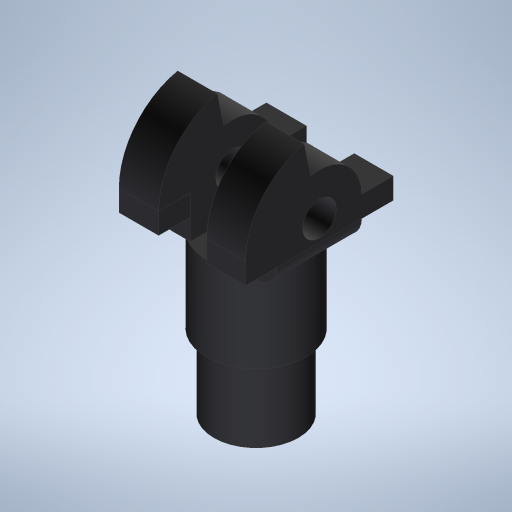
# Autodesk Inventor part: hingejoint2
Saved by Autodesk Inventor 2024 (Build 280153000, 153)
## iProperties
Created: 2024-05-16
Part Number: hingejoint2
Material: Generic
Document SubType Name: Modeling
Designer: maja6
Density: 1 g/cm^3
Appearance: Default
Author: maja6
Autodesk Inventor part; units mm, degrees
ref_plane "YZ Plane" through (0, 0, 0) normal (1, 0, 0) x (0, 1, 0)
ref_plane "XZ Plane" through (0, 0, 0) normal (0, 1, 0) x (-1, 0, 0)
ref_plane "XY Plane" through (0, 0, 0) normal (0, 0, 1) x (1, 0, 0)
sketch "Sketch1" plane through (0, 0, 0) normal (0, 0, 1) x (1, 0, 0)
  circle A0 centre (0, 0) radius 2
  circle A1 centre (0, 0) radius 4
  dimension "d0" = 4
  dimension "d1" = 8
  constraints: 2 centre point, 2 coincident
  measures "d0" diameter of A0
  measures "d1" diameter of A1
extrude "Extrusion1" add sketch "Sketch1" along normal blind 15
sketch "Sketch2" plane through (0, 0, 15) normal (0, 0, 1) x (1, 0, 0)
  circle A0 centre (0, 0) radius 4 projected
  line L0 (0, 4) -> (6, 4)
  line L1 (6, 4) -> (6, -4)
  line L2 (6, -4) -> (0, -4)
  line L3 (0, -4) -> (0, 4)
  line L4 (0, 4) -> (-6, 4)
  line L5 (-6, 4) -> (-6, -4)
  line L6 (-6, -4) -> (0, -4)
  line L7 (0, -4) -> (0, 4)
  dimension "d4" = 6
  dimension "d5" = 6
  constraints: 16 end point, 4 parallel, 2 horizontal, 2 perpendicular, 1 point on line, 1 vertical alignment, 1 other
  measures "d4" distance of L1.end L2.end
  measures "d5" distance of L6.end L5.end
extrude "Extrusion2" add sketch "Sketch2" along normal blind 8
sketch "Sketch3" plane through (0, 0, 23) normal (0, 0, 1) x (1, 0, 0)
  line L0 (6, 4) -> (-6, 4) projected
  line L1 (-6, -4) -> (6, -4) projected
  line L2 (-2.2377, 4) -> (2.306, 4)
  line L3 (2.306, 4) -> (2.306, -4)
  line L4 (2.306, -4) -> (-2.2377, -4)
  line L5 (-2.2377, -4) -> (-2.2377, 4)
  point P0 (0, 0)
  constraints: 8 end point, 2 parallel, 2 point on line, 1 horizontal, 1 perpendicular
extrude "Extrusion3" cut sketch "Sketch3" against normal blind 8
sketch "Sketch4" plane through (0, 0, 15) normal (0, 0, -1) x (-1, 0, 0)
  circle A0 centre (0, 0) radius 4
  circle A1 centre (0, 0) radius 4.731
  constraints: 2 centre point, 2 coincident
extrude "Extrusion4" add sketch "Sketch4" along normal blind 8
sketch "Sketch5" plane through (6, -4, 15) normal (1, 0, 0) x (0, 0, -1)
  line L0 (0, 8) -> (-8, 8) projected
  line L1 (0, 0) -> (-8, 0) projected
  line L2 (-8, 8) -> (0, 8)
  line L3 (0, 8) -> (0, 0)
  line L4 (0, 0) -> (-8, 0)
  line L5 (-8, 0) -> (-8, 8)
  circle A0 centre (-4, 4) radius 1.6
  circle A1 centre (-4, 4) radius 4
  point P0 (15, 4)
  point P1 (-8, 4)
  point P2 (-4, 8)
  point P3 (-4, 0)
  dimension "d12" = 3.2
  constraints: 8 end point, 2 centre point, 2 parallel, 1 coincident, 1 horizontal, 1 perpendicular
  measures "d12" diameter of A0
extrude "Extrusion5" cut sketch "Sketch5" against normal blind 14 contours A1 L5 L0 | A1 L1 L5 | A0
fillet "Fillet1" radius 2 2 edges at (-6, 0, 15) (6, 0, 15)
sketch "Sketch7" plane through (2.306, 4, 15) normal (0, 1, 0) x (1, 0, 0)
  point P0 (-2.306, 15)
sketch "Sketch8" plane through (2.306, 4, 15) normal (0, 1, 0) x (1, 0, 0)
  line L0 (0, -4) -> (3.694, -4) projected
  line L1 (0, 0) -> (0, -4) projected
  line L2 (3.694, -4) -> (0, -4)
  line L3 (0, -4) -> (0, -2)
  line L4 (0, -2) -> (3.694, -2)
  line L5 (3.694, -2) -> (3.694, -4)
  line L6 (-4.5455, -4) -> (-8.3301, -4)
  line L7 (-8.3301, -4) -> (-8.3301, -2)
  line L8 (-8.3301, -2) -> (-4.5455, -2)
  line L9 (-4.5455, -2) -> (-4.5455, -4)
  point P0 (-2.306, 15)
  constraints: 16 end point, 4 parallel, 2 horizontal, 2 perpendicular, 2 point on line, 1 midpoint
extrude "Extrusion7" add sketch "Sketch8" along normal blind 3
sketch "Sketch9" plane through (-2.5263, -4, 15) normal (0, -1, 0) x (1, 0, 0)
  line L0 (-3.4737, 2) -> (-3.4737, 4) projected
  line L1 (0.2868, 2) -> (-3.4978, 2) projected
  line L2 (-3.4737, 4) -> (0.2868, 4)
  line L3 (0.2868, 4) -> (0.2868, 2)
  line L4 (0.2868, 2) -> (-3.4737, 2)
  line L5 (-3.4737, 2) -> (-3.4737, 4)
  line L6 (4.8006, 4) -> (8.5263, 4)
  line L7 (8.5263, 4) -> (8.5263, 2)
  line L8 (8.5263, 2) -> (4.8006, 2)
  line L9 (4.8006, 2) -> (4.8006, 4)
  point P0 (2.5263, -15)
  constraints: 16 end point, 4 parallel, 2 horizontal, 2 perpendicular, 2 point on line
extrude "Extrusion8" add sketch "Sketch9" along normal blind 3
sketch "Sketch10" plane through (6, 4, 17) normal (1, 0, 0) x (0, 0, -1)
  circle A0 centre (-1.9999, -4) radius 7
  circle A1 centre (-2, -4) radius 1.6 projected
  circle A2 centre (-2, -4) radius 4
  line L0 (-2, -8) -> (-1.9999, -11)
  line L1 (-2, -4) -> (-8.8503, -5.4392)
  point P0 (17, -4)
  point P1 (-5.9145, -4.8224)
  dimension "d24" = 14
  constraints: 4 end point, 2 point on circle, 1 centre point, 1 coincident, 3 other
  measures "d24" diameter of A0
extrude "Extrusion9" add sketch "Sketch10" against normal blind 12 contours L1 A2 L0 A0 picked at (-2.5257, -9.94)
sketch "Sketch11" plane through (-2.5263, -4, 15) normal (0, -1, 0) x (1, 0, 0)
  line L0 (0, 0) -> (0.2886, 0) projected
  line L1 (0.2886, 0) -> (4.8323, 0)
  line L2 (4.8323, 0) -> (4.8323, 13.1536)
  line L3 (4.8323, 13.1536) -> (0.2886, 13.1536)
  line L4 (0.2886, 13.1536) -> (0.2886, 0)
  point P0 (2.5263, -15)
  constraints: 8 end point, 2 parallel, 1 horizontal, 1 perpendicular
extrude "Extrusion10" cut sketch "Sketch11" along normal mid plane 12
sketch "Sketch12" plane through (0, 0, 0) normal (0, 0, -1) x (-1, 0, 0)
  circle A0 centre (0, 0) radius 2.075
  dimension "d29" = 4.15
  constraints: 1 centre point, 1 coincident
  measures "d29" diameter of A0
extrude "Extrusion11" cut sketch "Sketch12" against normal blind 20
sketch "Sketch13" plane through (0, 0, 15) normal (0, 0, 1) x (1, 0, 0)
  circle A0 centre (0, 0) radius 2.2168
  constraints: 1 centre point, 1 coincident
extrude "Extrusion12" add sketch "Sketch13" against normal blind 1
body "Solid1"
